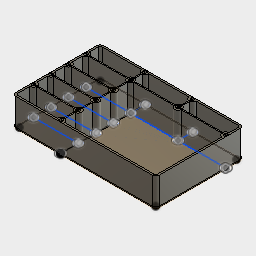
SIK_inserts v8 (Autodesk Fusion 360 design; units mm, degrees)
Autodesk Fusion 360 part; units mm, degrees
sketch "Sketch1" plane through (0, 0, 0) normal (0, 1, 0) x (1, 0, 0)
  line L0 (-107.65, -65.5) -> (133.65, -65.5)
  line L1 (140, -59.15) -> (140, 83.725)
  line L2 (133.65, 90.075) -> (-107.65, 90.075)
  line L3 (-114, 83.725) -> (-114, -59.15)
  arc A0 (-114, -59.15) -> (-107.65, -65.5) centre (-107.65, -59.15) ccw
  arc A1 (140, 83.725) -> (133.65, 90.075) centre (133.65, 83.725) ccw
  arc A2 (133.65, -65.5) -> (140, -59.15) centre (133.65, -59.15) ccw
  arc A3 (-107.65, 90.075) -> (-114, 83.725) centre (-107.65, 83.725) ccw
  point P0 (-114, -65.5)
  point P1 (140, -65.5)
  point P2 (-114, 90.075)
  dimension "d1" = 155.575
  dimension "d2" = 254
  dimension "d3" = 6.35
  dimension "d4" = 6.35
  dimension "d5" = 6.35
  dimension "d6" = 6.35
  measures "d1" distance of P0 P2
  measures "d2" distance of P0 P1
  measures "d3" radius of A0
  measures "d4" radius of A1
  measures "d5" radius of A2
  measures "d6" radius of A3
extrude "Extrude1" add sketch "Sketch1" along normal blind 3.175 makes body 1
sketch "Sketch2" plane through (0, 3.175, 0) normal (0, 1, 0) x (-1, 0, 0)
  arc A0 (107.65, -90.075) -> (114, -83.725) centre (107.65, -83.725) ccw
  line L0 (114, -83.725) -> (114, 59.15)
  arc A1 (114, 59.15) -> (107.65, 65.5) centre (107.65, 59.15) ccw
  line L1 (107.65, 65.5) -> (-133.65, 65.5)
  arc A2 (-133.65, 65.5) -> (-140, 59.15) centre (-133.65, 59.15) ccw
  line L2 (-140, 59.15) -> (-140, -83.725)
  arc A3 (-140, -83.725) -> (-133.65, -90.075) centre (-133.65, -83.725) ccw
  line L3 (-133.65, -90.075) -> (107.65, -90.075)
  line L4 (-136.825, 59.15) -> (-136.825, -83.725)
  arc A4 (-136.825, -83.725) -> (-133.65, -86.9) centre (-133.65, -83.725) ccw
  line L5 (-133.65, -86.9) -> (107.65, -86.9)
  arc A5 (107.65, -86.9) -> (110.825, -83.725) centre (107.65, -83.725) ccw
  line L6 (110.825, -83.725) -> (110.825, 59.15)
  arc A6 (110.825, 59.15) -> (107.65, 62.325) centre (107.65, 59.15) ccw
  line L7 (107.65, 62.325) -> (-133.65, 62.325)
  arc A7 (-133.65, 62.325) -> (-136.825, 59.15) centre (-133.65, 59.15) ccw
  circle A8 centre (31.45, 62.325) radius 3.175
  circle A9 centre (-136.825, -61.5) radius 3.175
  circle A10 centre (31.45, -61.5) radius 3.175
  circle A11 centre (31.45, -86.9) radius 3.175
  circle A12 centre (110.825, -61.5) radius 3.175
  circle A13 centre (31.45, 31.3688) radius 3.175
  circle A14 centre (31.45, 0.4125) radius 3.175
  circle A15 centre (31.45, -30.5437) radius 3.175
  circle A16 centre (-52.6875, -61.5) radius 3.175
  circle A17 centre (-52.6875, -86.9) radius 3.175
  circle A18 centre (110.825, -30.5437) radius 3.175
  circle A19 centre (110.825, 0.4125) radius 3.175
  circle A20 centre (110.825, 31.3688) radius 3.175
  circle A21 centre (31.45, 62.325) radius 6.35
  circle A22 centre (31.45, 31.3688) radius 6.35
  circle A23 centre (31.45, 0.4125) radius 6.35
  circle A24 centre (110.825, 31.3688) radius 6.35
  circle A25 centre (110.825, 0.4125) radius 6.35
  circle A26 centre (31.45, -30.5437) radius 6.35
  circle A27 centre (110.825, -30.5437) radius 6.35
  circle A28 centre (110.825, -61.5) radius 6.35
  circle A29 centre (31.45, -61.5) radius 6.35
  circle A30 centre (31.45, -86.9) radius 6.35
  circle A31 centre (-52.6875, -86.9) radius 6.35
  circle A32 centre (-52.6875, -61.5) radius 6.35
  circle A33 centre (-136.825, -61.5) radius 6.35
  line L8 (31.45, 31.3688) -> (110.825, 31.3688)
  line L9 (31.45, 0.4125) -> (110.825, 0.4125)
  line L10 (31.45, -30.5437) -> (110.825, -30.5437)
  line L11 (31.45, -61.5) -> (110.825, -61.5)
  line L12 (-52.6875, -61.5) -> (31.45, -61.5)
  line L13 (-136.825, -61.5) -> (-52.6875, -61.5)
  line L14 (-52.6875, -86.9) -> (-52.6875, -61.5)
  line L15 (31.45, -86.9) -> (31.45, -61.5)
  line L16 (31.45, -61.5) -> (31.45, -30.5437)
  line L17 (31.45, 0.4125) -> (31.45, -30.5437)
  line L18 (31.45, 31.3688) -> (31.45, 0.4125)
  line L19 (31.45, 62.325) -> (31.45, 31.3688)
  line L20 (31.45, 62.325) -> (31.45, 31.3688)
  line L21 (30.45, 62.325) -> (30.45, 31.3688)
  line L22 (31.45, 62.325) -> (31.45, 31.3688)
  line L23 (31.45, 62.325) -> (31.45, 31.3688)
  line L24 (32.45, 62.325) -> (32.45, 31.3688)
  line L25 (32.45, 31.3688) -> (32.45, 0.4125)
  line L26 (30.45, 31.3688) -> (30.45, 0.4125)
  line L27 (32.45, 0.4125) -> (32.45, -30.5437)
  line L28 (30.45, 0.4125) -> (30.45, -33.5572)
  line L29 (32.45, -30.5437) -> (32.45, -61.5)
  line L30 (30.45, -31.6976) -> (30.45, -61.5)
  line L31 (32.45, -61.5) -> (32.45, -86.9)
  line L32 (30.45, -61.5) -> (30.45, -86.9)
  line L33 (31.45, 30.3688) -> (110.825, 30.3688)
  line L34 (31.45, 31.3688) -> (110.825, 31.3688)
  line L35 (31.45, 32.3688) -> (110.825, 32.3688)
  line L36 (31.45, -0.5875) -> (110.825, -0.5875)
  line L37 (31.45, 0.4125) -> (110.825, 0.4125)
  line L38 (31.45, 1.4125) -> (110.825, 1.4125)
  line L39 (31.45, -31.5437) -> (110.825, -31.5437)
  line L40 (31.45, -30.5437) -> (110.825, -30.5437)
  line L41 (31.45, -29.5437) -> (110.825, -29.5437)
  line L42 (110.825, -61.5) -> (31.45, -61.5)
  line L43 (110.825, -60.5) -> (31.45, -60.5)
  line L44 (110.825, -62.5) -> (31.45, -62.5)
  line L45 (31.45, -62.5) -> (-136.825, -62.5)
  line L46 (31.45, -60.5) -> (-136.825, -60.5)
  line L47 (-52.6875, -61.5) -> (-52.6875, -86.9)
  line L48 (-51.6875, -86.9) -> (-51.6875, -61.5)
  line L49 (-53.6875, -86.9) -> (-53.6875, -61.5)
  line L50 (-133.65, -88.575) -> (107.65, -88.575)
  arc A34 (107.65, -88.575) -> (112.5, -83.725) centre (107.65, -83.725) ccw
  line L51 (112.5, -83.725) -> (112.5, 59.15)
  arc A35 (112.5, 59.15) -> (107.65, 64) centre (107.65, 59.15) ccw
  line L52 (107.65, 64) -> (-133.65, 64)
  arc A36 (-133.65, 64) -> (-138.5, 59.15) centre (-133.65, 59.15) ccw
  line L53 (-138.5, 59.15) -> (-138.5, -83.725)
  arc A37 (-138.5, -83.725) -> (-133.65, -88.575) centre (-133.65, -83.725) ccw
  line L54 (-136.825, -61.5) -> (-134.5799, -63.7451)
  line L55 (-136.825, -61.5) -> (-133.65, -61.5) construction
  line L56 (-136.825, -61.5) -> (-139.0701, -59.2549)
  line L57 (-136.825, -61.5) -> (-133.65, -61.5) construction
  line L58 (-136.825, -61.5) -> (-139.0701, -63.7451)
  line L59 (-136.825, -61.5) -> (-134.5799, -59.2549)
  line L60 (-136.4714, -61.8536) -> (-134.2264, -59.6085)
  line L61 (-136.4714, -61.8536) -> (-138.7165, -64.0986)
  line L62 (-139.0701, -63.7451) -> (-134.5799, -59.2549)
  line L63 (-139.4236, -63.3915) -> (-134.9335, -58.9014)
  line L64 (-136.4714, -61.1464) -> (-134.2264, -63.3915)
  line L65 (-136.4714, -61.1464) -> (-138.7165, -58.9014)
  line L66 (-134.5799, -63.7451) -> (-139.0701, -59.2549)
  line L67 (-134.9335, -64.0986) -> (-139.4236, -59.6085)
  line L68 (-136.4714, -61.8536) -> (-138.7165, -64.0986)
  line L69 (-139.4236, -63.3915) -> (-134.9335, -58.9014)
  line L70 (-136.4714, -61.1464) -> (-138.7165, -58.9014)
  line L71 (-136.4714, -61.8536) -> (-134.2264, -59.6085)
  line L72 (-136.4714, -61.1464) -> (-134.2264, -63.3915)
  circle A38 centre (-136.825, -61.5) radius 3.175
  line L73 (-50.796, -64.0986) -> (-55.2861, -59.6085)
  line L74 (-52.3339, -61.1464) -> (-54.579, -58.9014)
  line L75 (-52.3339, -61.1464) -> (-50.0889, -63.3915)
  line L76 (-52.3339, -61.8536) -> (-54.579, -64.0986)
  line L77 (-55.2861, -63.3915) -> (-50.796, -58.9014)
  line L78 (-52.3339, -61.8536) -> (-50.0889, -59.6085)
  circle A39 centre (-52.6875, -61.5) radius 3.175
  line L79 (-55.2861, -88.7915) -> (-50.796, -84.3014)
  line L80 (-52.3339, -87.2536) -> (-54.579, -89.4986)
  circle A40 centre (-52.6875, -86.9) radius 3.175
  line L81 (-50.796, -89.4986) -> (-55.2861, -85.0085)
  line L82 (-52.3339, -86.5464) -> (-50.0889, -88.7915)
  line L83 (-52.3339, -87.2536) -> (-50.0889, -85.0085)
  line L84 (-52.3339, -86.5464) -> (-54.579, -84.3014)
  line L85 (28.8514, -63.3915) -> (33.3415, -58.9014)
  line L86 (31.8036, -61.8536) -> (29.5585, -64.0986)
  circle A41 centre (31.45, -61.5) radius 3.175
  line L87 (33.3415, -64.0986) -> (28.8514, -59.6085)
  line L88 (31.8036, -61.1464) -> (34.0486, -63.3915)
  line L89 (31.8036, -61.8536) -> (34.0486, -59.6085)
  line L90 (31.8036, -61.1464) -> (29.5585, -58.9014)
  line L91 (28.8514, -88.7915) -> (33.3415, -84.3014)
  line L92 (31.8036, -87.2536) -> (29.5585, -89.4986)
  circle A42 centre (31.45, -86.9) radius 3.175
  line L93 (33.3415, -89.4986) -> (28.8514, -85.0085)
  line L94 (31.8036, -86.5464) -> (34.0486, -88.7915)
  line L95 (31.8036, -87.2536) -> (34.0486, -85.0085)
  line L96 (31.8036, -86.5464) -> (29.5585, -84.3014)
  line L97 (108.2264, -63.3915) -> (112.7165, -58.9014)
  line L98 (111.1786, -61.8536) -> (108.9335, -64.0986)
  circle A43 centre (110.825, -61.5) radius 3.175
  line L99 (112.7165, -64.0986) -> (108.2264, -59.6085)
  line L100 (111.1786, -61.1464) -> (113.4236, -63.3915)
  line L101 (111.1786, -61.8536) -> (113.4236, -59.6085)
  line L102 (111.1786, -61.1464) -> (108.9335, -58.9014)
  line L103 (28.8514, -32.4353) -> (33.3415, -27.9451)
  line L104 (31.8036, -30.8973) -> (29.5585, -33.1424)
  circle A44 centre (31.45, -30.5437) radius 3.175
  line L105 (33.3415, -33.1424) -> (28.8514, -28.6522)
  line L106 (31.8036, -30.1902) -> (34.0486, -32.4353)
  line L107 (31.8036, -30.8973) -> (34.0486, -28.6522)
  line L108 (31.8036, -30.1902) -> (29.5585, -27.9451)
  line L109 (28.8514, -1.479) -> (33.3415, 3.0111)
  line L110 (31.8036, 0.0589) -> (29.5585, -2.1861)
  circle A45 centre (31.45, 0.4125) radius 3.175
  line L111 (33.3415, -2.1861) -> (28.8514, 2.304)
  line L112 (31.8036, 0.7661) -> (34.0486, -1.479)
  line L113 (31.8036, 0.0589) -> (34.0486, 2.304)
  line L114 (31.8036, 0.7661) -> (29.5585, 3.0111)
  line L115 (108.2264, -32.4353) -> (112.7165, -27.9451)
  line L116 (111.1786, -30.8973) -> (108.9335, -33.1424)
  circle A46 centre (110.825, -30.5437) radius 3.175
  line L117 (112.7165, -33.1424) -> (108.2264, -28.6522)
  line L118 (111.1786, -30.1902) -> (113.4236, -32.4353)
  line L119 (111.1786, -30.8973) -> (113.4236, -28.6522)
  line L120 (111.1786, -30.1902) -> (108.9335, -27.9451)
  line L121 (108.2264, -1.479) -> (112.7165, 3.0111)
  line L122 (111.1786, 0.0589) -> (108.9335, -2.1861)
  circle A47 centre (110.825, 0.4125) radius 3.175
  line L123 (112.7165, -2.1861) -> (108.2264, 2.304)
  line L124 (111.1786, 0.7661) -> (113.4236, -1.479)
  line L125 (111.1786, 0.0589) -> (113.4236, 2.304)
  line L126 (111.1786, 0.7661) -> (108.9335, 3.0111)
  line L127 (28.8514, 29.4772) -> (33.3415, 33.9674)
  line L128 (31.8036, 31.0152) -> (29.5585, 28.7701)
  circle A48 centre (31.45, 31.3688) radius 3.175
  line L129 (33.3415, 28.7701) -> (28.8514, 33.2603)
  line L130 (31.8036, 31.7223) -> (34.0486, 29.4772)
  line L131 (31.8036, 31.0152) -> (34.0486, 33.2603)
  line L132 (31.8036, 31.7223) -> (29.5585, 33.9674)
  line L133 (108.2264, 29.4772) -> (112.7165, 33.9674)
  line L134 (111.1786, 31.0152) -> (108.9335, 28.7701)
  circle A49 centre (110.825, 31.3688) radius 3.175
  line L135 (112.7165, 28.7701) -> (108.2264, 33.2603)
  line L136 (111.1786, 31.7223) -> (113.4236, 29.4772)
  line L137 (111.1786, 31.0152) -> (113.4236, 33.2603)
  line L138 (111.1786, 31.7223) -> (108.9335, 33.9674)
  line L139 (28.8514, 60.4335) -> (33.3415, 64.9236)
  line L140 (31.8036, 61.9714) -> (29.5585, 59.7264)
  circle A50 centre (31.45, 62.325) radius 3.175
  line L141 (33.3415, 59.7264) -> (28.8514, 64.2165)
  line L142 (31.8036, 62.6786) -> (34.0486, 60.4335)
  line L143 (31.8036, 61.9714) -> (34.0486, 64.2165)
  line L144 (31.8036, 62.6786) -> (29.5585, 64.9236)
  point P0 (31.45, -61.5)
  dimension "d9" = 3.175
  dimension "d12" = 165.1
  dimension "d13" = 120.65
  dimension "d14" = 6.35
  dimension "d15" = 6.35
  dimension "d18" = 6.35
  dimension "d19" = 6.35
  dimension "d20" = 6.35
  dimension "d21" = 6.35
  dimension "d22" = 6.35
  dimension "d23" = 6.35
  dimension "d24" = 6.35
  dimension "d25" = 6.35
  dimension "d26" = 6.35
  dimension "d27" = 6.35
  dimension "d28" = 6.35
  dimension "d29" = 3.175
  dimension "d30" = 3.175
  dimension "d31" = 3.175
  dimension "d32" = 3.175
  dimension "d33" = 3.175
  dimension "d34" = 3.175
  dimension "d35" = 3.175
  dimension "d36" = 3.175
  dimension "d37" = 3.175
  dimension "d38" = 3.175
  dimension "d39" = 3.175
  dimension "d40" = 3.175
  dimension "d41" = 3.175
  dimension "d42" = 1
  dimension "d43" = 1
  dimension "d44" = 1
  dimension "d45" = 1
  dimension "d46" = 1
  dimension "d47" = 1
  dimension "d48" = 1
  dimension "d49" = 1
  dimension "d50" = 1
  dimension "d51" = 1
  dimension "d52" = 1
  dimension "d53" = 1
  dimension "d54" = 1.5
  dimension "d58" = 45
  dimension "d59" = 135
  dimension "d60" = 0.5
  dimension "d61" = 0.5
  dimension "d62" = 0.5
  dimension "d63" = 0.5
  dimension "d64" = 6.35
  dimension "d65" = 6.35
  dimension "d66" = 6.35
  dimension "d67" = 6.35
  dimension "d68" = 6.35
  dimension "d69" = 6.35
  dimension "d70" = 6.35
  dimension "d71" = 6.35
  dimension "d72" = 6.35
  dimension "d73" = 6.35
  dimension "d74" = 6.35
  dimension "d75" = 6.35
  dimension "d76" = 6.35
  measures "d12" distance of L7.end A8.centre
  measures "d13" distance of L4.start A9.centre
  measures "d14" diameter of A8
  measures "d15" diameter of A9
  measures "d18" diameter of A10
  measures "d19" diameter of A11
  measures "d20" diameter of A12
  measures "d21" diameter of A13
  measures "d22" diameter of A14
  measures "d23" diameter of A15
  measures "d24" diameter of A16
  measures "d25" diameter of A17
  measures "d26" diameter of A18
  measures "d27" diameter of A19
  measures "d28" diameter of A20
  measures "d29" distance of A8
  measures "d30" distance of A13
  measures "d31" distance of A14
  measures "d32" distance of A20
  measures "d33" distance of A19
  measures "d34" distance of A15
  measures "d35" distance of A18
  measures "d36" distance of A12
  measures "d37" distance of A10
  measures "d38" distance of A11
  measures "d39" distance of A17
  measures "d40" distance of A16
  measures "d41" distance of A9
  measures "d58" angle of L54 L55
  measures "d59" angle of L56 L57
  measures "d64" diameter of A38
  measures "d65" diameter of A39
  measures "d66" diameter of A40
  measures "d67" diameter of A41
  measures "d68" diameter of A42
  measures "d69" diameter of A43
  measures "d70" diameter of A44
  measures "d71" diameter of A45
  measures "d72" diameter of A46
  measures "d73" diameter of A47
  measures "d74" diameter of A48
  measures "d75" diameter of A49
  measures "d76" diameter of A50
extrude "Extrude2" add sketch "Sketch2" along normal blind 50.8 contours A0 L0 L3 A28 A30 L50 A34 L51 | L3 A11 A30 L50 A42 | L0 A12 A28 L51 A43 | L3 A11 A30 L50 A42 | A11 L50 L92 A42 L93 | L3 A30 A31 L50 | L5 A11 A30 L50 A42 | L5 A5 L6 A28 A30 L50 A34 L51 | L0 A12 A28 L51 A43 | A12 L51 A43 L100 L101 | L6 A12 A28 L51 A43 | A11 L50 L91 L92 A42 | A11 L50 A42 L93 L94 | L3 A17 A31 L50 A40 | L5 A30 A31 L50 | L5 A11 A30 L50 A42 | L5 A11 A30 L31 A42 | A11 L50 A42 L94 | L0 A27 A28 L51 | A12 L51 L97 A43 L101 | A12 L51 A43 L99 L100 | L6 A12 A28 L44 A43 | A12 L51 A43 L99 | A11 L50 L91 A42 | L3 A17 A31 L50 A40 | A17 L50 L80 A40 L81 | L2 A3 L3 A31 A33 L50 L53 A37 | L5 A17 A31 L50 A40 | L5 A11 A30 L32 A42 | L0 A18 A27 L51 A46 | L6 A12 A28 L51 A43 | L6 A27 A28 L51 | A12 L51 L97 A43 | A17 L50 L79 L80 A40 | A17 L50 A40 L81 L82 | L4 A4 L5 A31 A33 L50 L53 A37 | L5 A17 A31 L50 A40 | L5 A17 A31 L48 A40 | A17 L50 A40 L82 | A10 A29 L31 L44 A41 | L0 A18 A27 L51 A46 | A18 L51 A46 L118 L119 | L6 A18 A27 L51 A46 | L6 A12 A28 L43 A43 | A17 L50 L79 A40 | L5 A17 A31 L49 A40 | A10 A29 L32 L45 A41 | L0 A25 A27 L51 | A18 L51 L115 A46 L119 | A18 L51 A46 L117 L118 | L6 A18 A27 L39 A46 | A18 L51 A46 L117 | L2 A9 A33 L53 A38 | A16 A32 L45 L48 A39 | L0 A19 A25 L51 A47 | L6 A18 A27 L51 A46 | L6 A25 A27 L51 | A18 L51 L115 A46 | A10 A29 L29 L43 A41 | L2 A9 A33 L53 A38 | A9 L53 L63 L67 L69 A38 | L1 A2 L2 A21 A33 L52 A36 L53 | L4 A9 A33 L53 A38 | A16 A32 L45 L49 A39 | L0 A19 A25 L51 A47 | A19 L51 A47 L124 L125 | L6 A19 A25 L51 A47 | L6 A18 A27 L41 A46 | A15 A26 L29 L39 A44 | A9 L53 L56 L66 L67 A38 | A9 L53 L58 L62 L63 L69 A38 | L4 L7 A7 A21 A33 L52 A36 L53 | L4 A9 A33 L53 A38 | L4 A9 A33 L45 A38 | A9 L53 L61 L68 A38 | A10 A29 L30 L46 A41 | L0 A24 A25 L51 | A19 L51 L121 A47 L125 | A19 L51 A47 L123 L124 | L6 A19 A25 L36 A47 | A19 L51 A47 L123 | A9 L53 L56 L65 L66 L70 A38 | A9 L53 L58 L61 L62 L68 A38 | L4 A9 A33 L46 A38 | A9 L53 L65 L70 A38 | A16 A32 L46 A39 | L0 A20 A24 L51 A49 | L6 A19 A25 L51 A47 | L6 A24 A25 L51 | A19 L51 L121 A47 | A15 A26 L27 L41 A44 | L1 A8 A21 L52 A50 | A15 A26 L28 L30 A44 | L0 A20 A24 L51 A49 | A20 L51 A49 L136 L137 | L6 A20 A24 L51 A49 | L6 A19 A25 L38 A47 | A14 A23 L27 L36 A45 | L1 A8 A21 L52 A50 | A8 L52 L139 A50 L144 | L0 A1 L1 A21 A24 L51 A35 L52 | L7 A8 A21 L52 A50 | A20 L51 L133 A49 L137 | A20 L51 A49 L135 L136 | L6 A20 A24 L33 A49 | A20 L51 A49 L135 | A8 L52 L139 A50 L143 | A8 L52 A50 L141 L144 | L6 A6 L7 A21 A24 L51 A35 L52 | L7 A8 A21 L52 A50 | L7 A8 A21 L21 A50 | A8 L52 A50 L141 | A14 A23 L26 L28 A45 | L6 A20 A24 L51 A49 | A20 L51 L133 A49 | A14 A23 L25 L38 A45 | A8 L52 A50 L143 | L7 A8 A21 L24 A50 | L6 A20 A24 L35 A49 | A13 A22 L25 L33 A48 | A13 A22 L21 L26 A48 | A13 A22 L24 L35 A48 bodies 1
fillet "Fillet1" radius 6.35 8 edges at (140, 0, -12.2875) (138.1401, 0, -88.2151) (13, 0, -90.075) (-112.1401, 0, -88.2151) (-114, 0, -12.2875) (-112.1401, 0, 63.6401) (13, 0, 65.5) (138.1401, 0, 63.6401) on bodies 1
extrude "Extrude3" add sketch "Sketch2" along normal blind 50.8 separate body contours A11 A30 L15 L31 A42 | A29 A30 L15 L31 | A29 A30 L15 L32 | A11 A30 L15 L32 A42 | A10 A29 L15 L31 A41 | A11 L15 L31 L91 A42 | A11 L31 L91 A42 | A17 A31 L14 L47 L48 A40 | A31 A32 L14 L47 L48 | A10 A29 L15 L32 A41 | A11 L32 A42 L96 | A11 L15 L32 A42 L96 | A10 L31 A41 L87 | A10 L15 L31 L44 A41 L87 | A31 A32 L14 L47 L49 | A17 A31 L14 L47 L49 A40 | A17 L14 L47 L48 L79 A40 | A17 L48 L79 A40 | A16 A32 L14 L47 L48 A39 | A29 A32 L12 L45 | A10 A29 L12 L45 A41 | A10 L15 L32 L45 L86 A41 | A10 L32 L86 A41 | A17 L49 A40 L84 | A17 L14 L47 L49 A40 L84 | A16 A32 L14 L47 L49 A39 | A16 A32 L12 L45 A39 | A16 L48 L73 A39 | A16 L14 L45 L47 L48 L73 A39 | A29 A32 L12 L46 | A10 A29 L12 L46 A41 | A10 L45 L85 A41 | A10 L12 L32 L45 L85 A41 | L15 L45 L86 | L15 L44 L87 | A32 A33 L13 L45 | A16 A32 L13 L45 A39 | A16 L14 L45 L47 L49 L76 A39 | A16 L49 L76 A39 | A16 A32 L12 L46 A39 | A16 L12 L45 L48 L75 A39 | A16 L45 L75 A39 | A10 L12 L30 L46 A41 L87 | A9 A33 L13 L45 A38 | A32 A33 L13 L46 | A16 A32 L13 L46 A39 | A16 L45 L77 A39 | A16 L13 L45 L49 L77 A39 | L14 L45 L47 L76 | L14 L45 L47 L73 | A16 L12 L46 L78 A39 | A10 L46 A41 L87 | L12 L30 L87 | L12 L32 L85 | A9 A33 L13 L46 A38 | A9 L13 L45 L64 L72 A38 | A9 L45 L64 L72 A38 | A16 L13 L46 L73 A39 | A16 L46 L78 A39 | L12 L48 L75 | A9 L46 L60 L71 A38 | A9 L13 L46 L60 L71 A38 | A16 L46 L73 A39 | L13 L49 L77 makes body 2 at (-2.3997, 20.1083, -60.5) makes body 3 at (-32.45, 37.0417, -77.4289) makes body 4 at (81.7378, 20.1083, -60.5) makes body 5 at (51.6875, 20.1083, -77.4289)
extrude "Extrude4" add sketch "Sketch2" along normal blind 50.8 separate body contours A28 A29 L11 L42 L44 | A12 A28 L11 L42 L44 A43 | A28 A29 L11 L42 L43 | A12 A28 L11 L42 L43 A43 | A12 L44 L97 A43 | A12 L11 L42 L44 L97 A43 | A10 A29 L11 L42 L44 A41 | A10 A29 L11 L42 L43 A41 | A12 L11 L42 L43 A43 L99 | A10 L11 L31 L42 L44 A41 L88 | A10 L44 A41 L88 | A12 L43 A43 L99 | A10 L11 L29 L42 L43 A41 L89 | A10 A29 L16 L29 A41 | A26 A29 L16 L29 | A10 L43 A41 L89 | L11 L31 L42 L88 | L11 L29 L42 L89 | A15 A26 L16 L29 A44 | A10 A29 L16 L30 A41 | A26 A29 L16 L30 | A10 L16 L29 L43 L85 A41 | A10 L29 L85 A41 | A15 A26 L16 L30 A44 | A15 L29 A44 L105 | A15 L16 L29 L39 A44 L105 | A10 L16 L30 L46 A41 L90 | A10 L30 A41 L90 | L16 L46 L90 | L16 L43 L85 | A15 L16 L28 L30 L104 A44 | A15 L28 L30 L104 A44 | L16 L39 L105 makes body 6 at (-83.3622, 20.1083, -60.5) makes body 7 at (-32.45, 37.0417, -41.867)
extrude "Extrude5" add sketch "Sketch2" along normal blind 50.8 separate body contours A26 A27 L10 L39 L40 | A18 A27 L10 L39 L40 A46 | A26 A27 L10 L40 L41 | A18 A27 L10 L40 L41 A46 | A18 L39 L115 A46 | A18 L10 L39 L40 L115 A46 | A18 L10 L40 L41 A46 L117 | A23 A25 L9 L36 L37 | A19 A25 L9 L36 L37 A47 | A18 L41 A46 L117 | A23 A25 L9 L37 L38 | A19 A25 L9 L37 L38 A47 | A14 A23 L9 L36 L37 A45 | A19 L36 L121 A47 | A19 L9 L36 L37 L121 A47 | A15 A26 L17 L27 A44 | A23 A26 L17 L27 | A23 A26 L17 L28 | A15 A26 L17 L28 A44 | A14 A23 L9 L37 L38 A45 | A19 L9 L37 L38 A47 L123 | A14 A23 L17 L27 A45 | A14 L9 L27 L36 L37 A45 L112 | A14 L36 A45 L112 | A15 L17 L27 L41 L103 A44 | A15 L27 L103 A44 | A14 A23 L17 L28 A45 | A15 L28 A44 L108 | A15 L17 L28 A44 L108 | A19 L38 A47 L123 | A14 L9 L25 L37 L38 A45 L113 | A14 L27 A45 L111 | A14 L17 L27 L36 A45 L111 | A14 L17 L28 L110 A45 | A14 L28 L110 A45 | A14 L38 A45 L113 | L9 L27 L37 L112 | L9 L25 L37 L113 | L17 L41 L103 | L17 L36 L111 makes body 8 at (-58.9128, 20.1083, -0.5875) makes body 9 at (-30.45, 20.1083, -10.9107) makes body 10 at (-61.0844, 20.1083, -31.5437)
extrude "Extrude6" add sketch "Sketch2" along normal blind 50.8 separate body contours A22 A24 L8 L33 L34 | A20 A24 L8 L33 L34 A49 | A8 A21 L19 L20 L21 L22 L23 A50 | A21 A22 L19 L20 L21 L22 L23 | A22 A23 L18 L26 | A14 A23 L18 L26 A45 | A22 A24 L8 L34 L35 | A20 A24 L8 L34 L35 A49 | A13 A22 L8 L33 L34 A48 | A20 L33 L133 A49 | A20 L8 L33 L34 L133 A49 | A14 A23 L18 L25 A45 | A22 A23 L18 L25 | A21 A22 L19 L20 L22 L23 L24 | A8 A21 L19 L20 L22 L23 L24 A50 | A8 L19 L20 L21 L22 L23 L140 A50 | A8 L21 L140 A50 | A13 A22 L19 L20 L21 L22 L23 A48 | A13 A22 L18 L26 A48 | A14 L26 A45 L114 | A14 L18 L26 A45 L114 | A13 A22 L8 L34 L35 A48 | A20 L8 L34 L35 A49 L135 | A13 A22 L18 L25 A48 | A13 L8 L25 L33 L34 A48 L130 | A13 L33 A48 L130 | A14 L18 L25 L38 L109 A45 | A14 L25 L109 A45 | A8 L24 A50 L141 | A8 L19 L20 L22 L23 L24 A50 L141 | A13 A22 L19 L20 L22 L23 L24 A48 | A13 L21 A48 L132 | A13 L19 L20 L21 L22 L23 A48 L132 | A13 L18 L26 L128 A48 | A13 L26 L128 A48 | A20 L35 A49 L135 | A13 L8 L24 L34 L35 A48 L131 | A13 L25 A48 L129 | A13 L18 L25 L33 A48 L129 | A13 L19 L20 L22 L23 L24 L35 L127 A48 | A13 L24 L127 A48 | L18 L38 L109 | A13 L35 A48 L131 | L8 L25 L34 L130 | L8 L24 L34 L131 | L19 L20 L22 L23 L35 L127 | L18 L33 L129 makes body 11 at (-32.45, 37.0417, 42.692) makes body 12 at (-58.9128, 37.0417, 30.3688) makes body 13 at (-32.45, 37.0417, 20.0455)
equation "d2 = 10\""
equation "d55 = 2\""
equation "d77 = 2\""
equation "d79 = 2\""
equation "d81 = 2\""
equation "d83 = 2\""
named bodies: "Tray"
